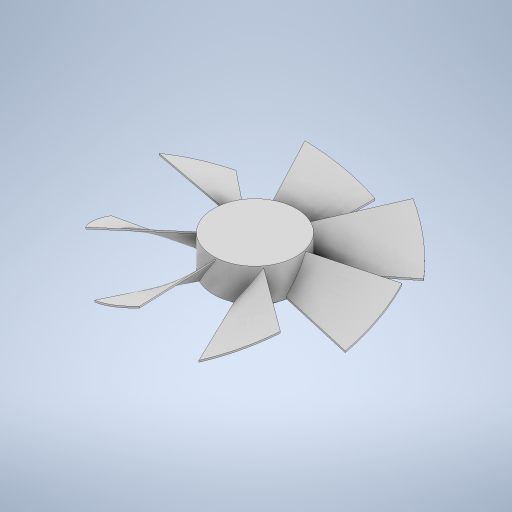
# Autodesk Inventor part: Ventoinha
Saved by Autodesk Inventor 2023.2 (Build 272271000, 271)
## iProperties
Created: 2022-12-15
Part Number: Ventoinha
Material: Generic
Document SubType Name: Sheet Metal
Designer: coqui
Density: 1 g/cm^3
Sheet Metal Rule: Default_mm
Appearance: Default
Author: coqui
Autodesk Inventor part; units mm, degrees
ref_plane "YZ Plane" through (0, 0, 0) normal (1, 0, 0) x (0, 1, 0)
ref_plane "XZ Plane" through (0, 0, 0) normal (0, 1, 0) x (-1, 0, 0)
ref_plane "XY Plane" through (0, 0, 0) normal (0, 0, 1) x (1, 0, 0)
sketch "Sketch1" plane through (0, 0, 0) normal (0, 0, 1) x (1, 0, 0)
  line L0 (0, 0) -> (0, 24)
  line L1 (0, 24) -> (25, 24)
  line L2 (25, 24) -> (25, 4)
  line L3 (25, 4) -> (20, 4)
  line L4 (20, 4) -> (20, 0)
  line L5 (20, 0) -> (0, 0)
  line L6 (0, -4.8611) -> (0, 32.7303) construction
  dimension "d0" = 25
  dimension "d1" = 20
  dimension "d2" = 4
  dimension "d4" = 5
  constraints: 14 end point, 5 perpendicular, 2 vertical
  measures "d0" distance of L0.end L1.end
  measures "d1" distance of L1.end L2.end
  measures "d2" distance of L3.end L4.end
  measures "d4" horizontal distance of L2.end L4.end
revolve "Revolution1" add sketch "Sketch1" angle 360 about axis through (0, -4.8611, 0) along (0, 1, 0)
sketch "Sketch9" plane through (0, 0, 0) normal (1, 0, 0) x (0, 1, 0)
  line L0 (0, 0) -> (-39.5663, 0) construction
  line L1 (4.5, -25) -> (5.5, -25)
  line L2 (5.5, -25) -> (5.5, -72.5)
  line L3 (5.5, -72.5) -> (4.5, -72.5)
  line L4 (4.5, -72.5) -> (4.5, -25)
  line L5 (0, -20) -> (0, 20) projected
  dimension "d28" = 1
  dimension "d29" = 25
  dimension "d30" = 4.5
  dimension "d31" = 47.5
  constraints: 10 end point, 2 horizontal, 2 parallel, 1 perpendicular
  measures "d28" distance of L1.start L1.end
  measures "d29" distance between parallel lines of L0 L1
  measures "d30" distance from line of L5 L1.start
  measures "d31" distance of L1.start L3.end
coil "Coil1" sketch "Sketch9" operation add axis through (0, 0, 0) along (0, 1, 0) pitch 226 turns 0.077434 hand right
pattern_circular "Circular Pattern1" count 7 over 360 about axis through (0, 14, 0) along (0, 1, 0) of "Coil1"
equation "\"BendRadius\" = Thickness"
equation "\"BendReliefWidth\" = Thickness"
equation "\"BendReliefDepth\" = 0.5 * Thickness"
equation "\"CornerReliefSize\" = 4 * Thickness"
equation "\"MinimumRemnant\" = 2 * Thickness"
equation "\"TransitionRadius\" = BendRadius"
equation "\"JacobiRadiusSize\" = BendRadius"
equation "\"GapSize\" = Thickness"
equation "\"Thickness\" = 0.5"
body "Solid1"
